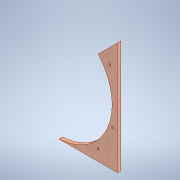
# Autodesk Inventor part: Hood (inside)
Saved by Autodesk Inventor 2020 (Build 240168000, 168)
## iProperties
Created: 2020-01-13
Part Number: Hood (inside)
Material: Wood (Oak)
Document SubType Name: Modeling
Designer: autum
Density: 0.76 g/cm^3
Appearance: White Oak - Natural Medium Gloss
Author: autum
Autodesk Inventor part; units mm, degrees
ref_plane "YZ Plane" through (0, 0, 0) normal (1, 0, 0) x (0, 1, 0)
ref_plane "XZ Plane" through (0, 0, 0) normal (0, 1, 0) x (-1, 0, 0)
ref_plane "XY Plane" through (0, 0, 0) normal (0, 0, 1) x (1, 0, 0)
sketch "Sketch1" plane through (0, 0, 0) normal (0, 0, 1) x (1, 0, 0)
  arc A0 (270.3829, -151.3678) -> (288.8718, 134.8752) centre (135.9788, 1.0322) ccw
  line L0 (358.2288, 204.2322) -> (358.2288, -202.1678)
  line L1 (358.2288, -202.1678) -> (147.3998, -202.1678)
  line L2 (147.3998, 204.2322) -> (553.7998, 204.2322) construction
  arc A1 (147.3998, -201.8466) -> (288.8718, 134.8752) centre (135.9788, 1.0322) ccw
  line L3 (147.3998, -201.8466) -> (147.3998, -202.1678)
  line L4 (358.2288, 204.2322) -> (288.8718, 134.8752)
  line L5 (358.2288, 204.2322) -> (456.3143, 204.2322) construction
  point P0 (270.3829, 153.4322)
  dimension "d5" = 203.2
  dimension "d9" = 135
  constraints: 12 end point, 4 point on circle, 2 centre point, 2 horizontal, 1 coincident, 1 equal length
  measures "d5" radius of A0
  measures "d9" angle of L4 L5
extrude "Extrusion1" add sketch "Sketch1" along normal blind 12.7
sketch "Sketch2" plane through (0, 0, 0) normal (0, 0, -1) x (-1, 0, 0)
  line L0 (-358.2288, -202.1678) -> (-358.2288, 204.2322) projected
  line L1 (-147.3998, -202.1678) -> (-358.2288, -202.1678) projected
  point P0 (0, 0)
  point P1 (-288.3788, -161.5278)
  point P2 (-341.7188, -68.8178)
  point P3 (-331.5588, 122.9522)
  dimension "d10" = 69.85
  dimension "d11" = 40.64
  dimension "d12" = 16.51
  dimension "d13" = 133.35
  dimension "d14" = 325.12
  dimension "d15" = 26.67
  measures "d10" distance from line of L0 point (-288.379, -161.528)
  measures "d11" distance from line of L1 point (-288.379, -161.528)
  measures "d12" distance from line of L0 point (-341.719, -68.818)
  measures "d13" vertical distance of L0.start point (-341.719, -68.818)
  measures "d14" distance from line of L1 point (-331.559, 122.952)
  measures "d15" distance from line of L0 point (-331.559, 122.952)
hole "Hole1" at (288.3788, -161.5278, 0) at (341.7188, -68.8178, 0) at (331.5588, 122.9522, 0) direction (0, 0, 1) diameter 6.7564 end through all
body "Solid1"
